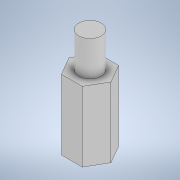
# Autodesk Inventor part: 10mmStandOff
Saved by Autodesk Inventor 2020 (Build 240168000, 168)
## iProperties
Created: 2019-08-05
Part Number: 10mmStandOff
Material: Generic
Document SubType Name: Modeling
Designer: n10208577
Density: 1 g/cm^3
Appearance: Default
Author: n10208577
Autodesk Inventor part; units mm, degrees
ref_plane "YZ Plane" through (0, 0, 0) normal (1, 0, 0) x (0, 1, 0)
ref_plane "XZ Plane" through (0, 0, 0) normal (0, 1, 0) x (-1, 0, 0)
ref_plane "XY Plane" through (0, 0, 0) normal (0, 0, 1) x (1, 0, 0)
sketch "Sketch1" plane through (0, 0, 0) normal (0, 1, 0) x (-1, 0, 0)
  circle A0 centre (0, 0) radius 1.6
  line L0 (0, 0) -> (3, 0)
  line L1 (3, 0) -> (1.5, -2.5981)
  line L2 (1.5, -2.5981) -> (-1.5, -2.5981)
  line L3 (-1.5, -2.5981) -> (-3, 0)
  line L4 (-3, 0) -> (-1.5, 2.5981)
  line L5 (-1.5, 2.5981) -> (1.5, 2.5981)
  line L6 (1.5, 2.5981) -> (3, 0)
  dimension "d0" = 3.2
  dimension "d1" = 3
  constraints: 14 end point, 2 coincident, 1 centre point, 1 horizontal, 13 other
  measures "d0" diameter of A0
  measures "d1" distance of L0.start L0.end
extrude "Extrusion1" add sketch "Sketch1" along normal blind 10
sketch "Sketch2" plane through (0, 10, 0) normal (0, 1, 0) x (1, 0, 0)
  circle A0 centre (0, 0) radius 1.6 projected
extrude "Extrusion2" add sketch "Sketch2" along normal blind 5 and the other way blind 2.5
body "Solid1"
